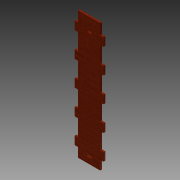
# Autodesk Inventor part: Panel3
Saved by Autodesk Inventor 2015 (Build 190159000, 159)
## iProperties
Created: 2014-08-06
Part Number: Panel3
Material: Wood (Oak)
Document SubType Name: Modeling
Designer: Patrick Camilleri
Density: 0.76 g/cm^3
Appearance: White Oak - Natural Medium Gloss
Author: Patrick Camilleri
Autodesk Inventor part; units mm, degrees
ref_plane "YZ Plane" through (0, 0, 0) normal (1, 0, 0) x (0, 1, 0)
ref_plane "XZ Plane" through (0, 0, 0) normal (0, 1, 0) x (-1, 0, 0)
ref_plane "XY Plane" through (0, 0, 0) normal (0, 0, 1) x (1, 0, 0)
sketch "Sketch1" plane through (0, 0, 0) normal (0, 1, 0) x (-1, 0, 0)
  line L0 (20, 120) -> (-20, 120)
  line L1 (-20, 120) -> (-20, -110.8)
  line L2 (-20, -110.8) -> (20, -110.8)
  line L3 (20, -110.8) -> (20, 120)
  line L4 (20, 0) -> (-20, 0) construction
  line L5 (0, -110.8) -> (0, 120) construction
  point P0 (0, 0)
  point P1 (0, 0)
  dimension "d57" = 40
  dimension "d58" = 110.8
  dimension "d59" = 120
  constraints: 12 end point, 3 midpoint, 2 parallel, 2 perpendicular, 2 point on line, 1 coincident, 1 horizontal
  measures "d57" distance of L1.end L2.end
  measures "d58" distance between parallel lines of L4 L2
  measures "d59" distance between parallel lines of L4 L0
extrude "Extrusion1" add sketch "Sketch1" along normal blind 3
sketch "Sketch3" plane through (0, 0, 0) normal (0, -1, 0) x (1, 0, 0)
  line L0 (-20, 120) -> (20, 120) projected
  line L1 (-20, -110.8) -> (-20, 120) projected
  line L2 (20, -110.8) -> (-20, -110.8) projected
  line L3 (20, 120) -> (20, -110.8) projected
  line L4 (-23, 123) -> (23, 123) construction
  line L5 (23, 123) -> (23, -113.8) construction
  line L6 (23, -113.8) -> (-23, -113.8) construction
  line L7 (-23, -113.8) -> (-23, 123) construction
  line L8 (-20, -110.8) -> (-20, 120) projected
  line L9 (-26, -78.9771) -> (-20, -78.9771)
  line L10 (-20, -78.9771) -> (-20, -93.9771)
  line L11 (-20, -93.9771) -> (-26, -93.9771)
  line L12 (-26, -93.9771) -> (-26, -78.9771)
  line L13 (-26, -78.9771) -> (-20, -93.9771) construction
  line L14 (-20, -78.9771) -> (-26, -93.9771) construction
  line L15 (26, -93.9771) -> (20, -93.9771)
  line L16 (20, -93.9771) -> (20, -78.9771)
  line L17 (20, -78.9771) -> (26, -78.9771)
  line L18 (26, -78.9771) -> (26, -93.9771)
  line L19 (26, -93.9771) -> (20, -78.9771) construction
  line L20 (20, -93.9771) -> (26, -78.9771) construction
  point P0 (0, 0)
  point P1 (-23, -86.4771)
  point P2 (23, -86.4771)
  dimension "d60" = 3
  dimension "d61" = 15
  dimension "d64" = 6
  dimension "d65" = 15
  constraints: 32 end point, 4 midpoint, 4 parallel, 3 point on line, 2 horizontal, 2 perpendicular, 3 other
  measures "d60" distance between parallel lines of L1 L7
  measures "d61" distance of L9.end L10.end
  measures "d64" distance of L16.end L17.end
  measures "d65" distance of L15.end L16.end
extrude "Extrusion3" add sketch "Sketch3" against normal blind 3 contours L1 L11 L12 L9 | L17 L18 L15 L3
pattern_linear "Rectangular Pattern1" count 5 spacing 45 along (0, 0, 1) of "Extrusion3"
sketch "Sketch4" plane through (0, 0, 0) normal (0, -1, 0) x (1, 0, 0)
  line L0 (20, -110.8) -> (-20, -110.8) projected
  line L1 (-4.15, -97.5) -> (4.15, -97.5)
  line L2 (4.15, -97.5) -> (4.15, -100.5)
  line L3 (4.15, -100.5) -> (-4.15, -100.5)
  line L4 (-4.15, -100.5) -> (-4.15, -97.5)
  line L5 (-4.15, -97.5) -> (4.15, -100.5) construction
  line L6 (4.15, -97.5) -> (-4.15, -100.5) construction
  point P0 (0, 0)
  point P1 (0, -99)
  dimension "d69" = 8.3
  dimension "d70" = 3
  dimension "d71" = 11.8
  constraints: 12 end point, 2 midpoint, 2 parallel, 1 horizontal, 1 perpendicular
  measures "d69" distance of L2.end L3.end
  measures "d70" distance of L1.end L2.end
  measures "d71" distance from line of L0 point (0, -99)
extrude "Extrusion4" cut sketch "Sketch4" against normal blind 3
pattern_linear "Rectangular Pattern2" count 2 spacing 195 along (0, 0, 1) of "Extrusion4"
body "Solid1"
